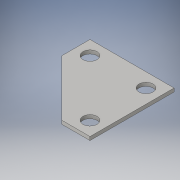
# Autodesk Inventor part: 3 inch gusset plate
Saved by Autodesk Inventor 2016 (Build 200138000, 138)
## iProperties
Created: 2016-02-04
Part Number: 3 inch gusset plate
Material: Generic
Document SubType Name: Modeling
Designer: gus
Density: 1 g/cm^3
Appearance: Default
Author: gus
Autodesk Inventor part; units mm, degrees
ref_plane "YZ Plane" through (0, 0, 0) normal (1, 0, 0) x (0, 1, 0)
ref_plane "XZ Plane" through (0, 0, 0) normal (0, 1, 0) x (-1, 0, 0)
ref_plane "XY Plane" through (0, 0, 0) normal (0, 0, 1) x (1, 0, 0)
sketch "Sketch1" plane through (0, 0, 0) normal (0, 1, 0) x (-1, 0, 0)
  line L0 (0, 0) -> (76.2, 0)
  line L1 (76.2, 0) -> (76.2, 25.4)
  line L2 (25.4, 76.2) -> (0, 76.2)
  line L3 (0, 76.2) -> (0, 0)
  line L4 (76.2, 25.4) -> (25.4, 76.2)
  circle A0 centre (63.5, 12.7) radius 6.35
  circle A1 centre (12.7, 63.5) radius 6.35
  circle A2 centre (12.7, 12.7) radius 6.35
  point P0 (76.2, 76.2)
  dimension "d0" = 76.2
  dimension "d1" = 76.2
  dimension "d2" = 50.8
  dimension "d3" = 50.8
  dimension "d4" = 12.7
  dimension "d5" = 12.7
  dimension "d6" = 12.7
  dimension "d7" = 12.7
  dimension "d8" = 50.8
  dimension "d9" = 50.8
  dimension "d10" = 12.7
  dimension "d11" = 12.7
  dimension "d12" = 12.7
  constraints: 10 end point, 3 centre point, 2 parallel, 2 point on line, 1 horizontal, 1 perpendicular
  measures "d0" distance of L2.end L0.start
  measures "d1" distance of L0.start L0.end
  measures "d2" distance of L1.end point (76.2, 76.2)
  measures "d3" distance of L2.start point (76.2, 76.2)
  measures "d4" diameter of A0
  measures "d5" diameter of A1
  measures "d6" diameter of A2
  measures "d7" distance from line of L1 A0.centre
  measures "d8" distance of A2.centre A0.centre
  measures "d9" distance of A1.centre A2.centre
  measures "d10" distance from line of L0 A0.centre
  measures "d11" distance from line of L3 A2.centre
  measures "d12" distance from line of L2 A1.centre
extrude "Extrusion1" add sketch "Sketch1" along normal blind 3.175
equation "\"d0\" = d1"
equation "\"d3\" = d2"
body "Solid1"
